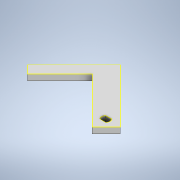
# Autodesk Inventor part: gripper (moving part
Saved by Autodesk Inventor 2020.1 (Build 241239000, 239)
## iProperties
Created: 2019-10-24
Part Number: gripper (moving part
Material: Generic
Document SubType Name: Modeling
Designer: amirs
Density: 1 g/cm^3
Appearance: Default
Author: amirs
Autodesk Inventor part; units mm, degrees
ref_plane "YZ Plane" through (0, 0, 0) normal (1, 0, 0) x (0, 1, 0)
ref_plane "XZ Plane" through (0, 0, 0) normal (0, 1, 0) x (-1, 0, 0)
ref_plane "XY Plane" through (0, 0, 0) normal (0, 0, 1) x (1, 0, 0)
sketch "Sketch1" plane through (0, 0, 0) normal (0, 1, 0) x (-1, 0, 0)
  line L0 (38.1169, -26.9408) -> (65.0577, -0.0001)
  line L1 (71.6583, -6.6007) -> (33.1013, -45.1577)
  line L2 (65.0577, -0.0001) -> (71.6583, -6.6007)
  circle A0 centre (0.0001, -0.0001) radius 0.88
  line L3 (2.525, 2.4129) -> (-2.5248, 2.4129)
  line L4 (2.525, -2.4131) -> (-2.5248, -2.4131)
  arc A1 (-2.5248, 2.4129) -> (-2.5248, -2.4131) centre (0.0001, -0.0001) ccw
  arc A2 (2.525, -2.4131) -> (2.525, 2.4129) centre (0.0001, -0.0001) ccw
  line L5 (38.1169, -26.9408) -> (-0.1838, 11.3598)
  line L6 (-0.1838, 11.3598) -> (-11.8, -0.2564)
  line L7 (33.1013, -45.1577) -> (-11.8, -0.2564)
  dimension "d12" = 1.76
  dimension "d14" = 4.826
  dimension "d17" = 63.5
  dimension "d25" = 3.4925
  constraints: 16 end point, 4 point on circle, 3 centre point, 2 horizontal, 2 perpendicular, 1 coincident, 1 parallel
  measures "d12" diameter of A0
  measures "d14" distance between parallel lines of L3 L4
  measures "d17" distance of L1.end L6.end
  measures "d25" radius of A2
extrude "Extrusion1" add sketch "Sketch1" along normal blind 5.08 contours L0 L2 L1 L7 L6 L5
sketch "Sketch2" plane through (0, 5.08, 0) normal (0, 1, 0) x (1, 0, 0)
  line L0 (-33.1013, 45.1577) -> (-71.6583, 6.6007) projected
  line L1 (-71.6583, 6.6007) -> (-65.0577, 0.0001) projected
  line L2 (-65.0577, 0.0001) -> (-38.1169, 26.9408) projected
  line L3 (-38.1169, 26.9408) -> (0.1838, -11.3598) projected
  line L4 (0.1838, -11.3598) -> (11.8, 0.2564) projected
  line L5 (11.8, 0.2564) -> (-33.1013, 45.1577) projected
  arc A0 (-2.525, 2.4131) -> (-2.525, -2.4129) centre (-0.0001, 0.0001) ccw projected
  line L6 (-2.525, 2.4131) -> (2.5248, 2.4131) projected
  arc A1 (2.5248, -2.4129) -> (2.5248, 2.4131) centre (-0.0001, 0.0001) ccw projected
  line L7 (2.5248, -2.4129) -> (-2.525, -2.4129) projected
  point P0 (0, 0)
body "Solid1"
